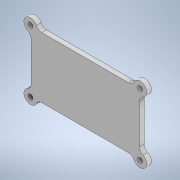
# Autodesk Inventor part: sensor_lid
Saved by Autodesk Inventor 2020 (Build 240168000, 168)
## iProperties
Created: 2020-03-10
Part Number: sensor_lid
Material: Generic
Document SubType Name: Modeling
Designer: Richard
Density: 1 g/cm^3
Appearance: Default
Author: Richard
Autodesk Inventor part; units mm, degrees
ref_plane "YZ Plane" through (0, 0, 0) normal (1, 0, 0) x (0, 1, 0)
sketch "Sketch1" plane through (0, 0, 0) normal (0, 0, 1) x (1, 0, 0)
  line L0 (-172.0273, 68.4234) -> (-119.9573, 68.4234)
  line L1 (-119.9573, 68.4234) -> (-119.9573, 42.0074)
  line L2 (-119.9573, 42.0074) -> (-172.0273, 42.0074)
  line L3 (-172.0273, 42.0074) -> (-172.0273, 68.4234)
  point P0 (0, 0)
  dimension "d0" = 52.07
  dimension "d1" = 26.416
  constraints: 8 end point, 2 parallel, 1 horizontal, 1 perpendicular
  measures "d0" distance of L1.end L2.end
  measures "d1" distance of L0.end L1.end
extrude "Extrusion1" add sketch "Sketch1" along normal blind 2.54
sketch "Sketch2" plane through (0, 0, 2.54) normal (0, 0, 1) x (1, 0, 0)
  line L0 (-119.9573, 68.4234) -> (-172.0273, 68.4234) projected
  line L1 (-119.9573, 68.4234) -> (-172.0273, 68.4234) projected
  line L2 (-172.0273, 68.4234) -> (-172.0273, 42.0074) projected
  line L3 (-172.0273, 42.0074) -> (-119.9573, 42.0074) projected
  line L4 (-119.9573, 42.0074) -> (-119.9573, 68.4234) projected
  line L5 (-116.7823, 38.8324) -> (-175.2023, 38.8324)
  line L6 (-175.2023, 38.8324) -> (-175.2023, 71.5984)
  line L7 (-175.2023, 71.5984) -> (-116.7823, 71.5984)
  line L8 (-116.7823, 71.5984) -> (-116.7823, 38.8324)
  point P0 (0, 0)
  dimension "d18" = 3.175
  dimension "d19" = 3.175
  dimension "d20" = 3.175
  dimension "d21" = 3.175
  dimension "d25" = 32.766
  dimension "d26" = 58.42
  constraints: 8 end point, 2 parallel, 1 horizontal, 1 perpendicular
  measures "d18" distance between parallel lines of L3 L5
  measures "d19" distance between parallel lines of L7 L0
  measures "d20" distance between parallel lines of L4 L8
  measures "d21" distance between parallel lines of L6 L2
  measures "d25" distance between parallel lines of L7 L5
  measures "d26" distance of L5.start L5.end
extrude "Extrusion2" add sketch "Sketch2" along normal blind 2.54 contours L4 L3 L2 L0 | L5 L6 L7 L8
fillet "Fillet1" radius 3.175 4 edges at (-116.7823, 38.8324, 3.81) (-175.2023, 38.8324, 3.81) (-116.7823, 71.5984, 3.81) (-175.2023, 71.5984, 3.81)
sketch "Sketch4" plane through (0, 0, 5.08) normal (0, 0, 1) x (1, 0, 0)
  circle A0 centre (-175.5648, 71.9609) radius 1.3891
  line L0 (-119.9573, 71.5984) -> (-172.0273, 71.5984) projected
  arc A1 (-172.0273, 71.5984) -> (-175.2023, 68.4234) centre (-172.0273, 68.4234) ccw projected
  line L1 (-175.2023, 68.4234) -> (-175.2023, 42.0074) projected
  arc A2 (-172.0273, 71.5984) -> (-175.2023, 68.4234) centre (-175.5648, 71.9609) ccw
  point P0 (0, 0)
  dimension "d12" = 2.7781
  dimension "d23" = 3.556
  constraints: 2 centre point, 2 point on circle, 1 concentric
  measures "d12" diameter of A0
  measures "d23" radius of A2
extrude "Extrusion3" add sketch "Sketch4" against normal up to surface (2.54 mm away)
ref_plane "Work Plane1" through (-145.9923, 42.0074, 2.54) normal (-1, 0, 0) x (0, 0, 1)
ref_plane "Work Plane2" through (-172.0273, 55.2154, 2.54) normal (0, -1, 0) x (1, 0, 0)
mirror "Mirror1" about plane through (-145.9923, 42.0074, 2.54) normal (-1, 0, 0) of "Extrusion3"
mirror "Mirror2" about plane through (-172.0273, 55.2154, 2.54) normal (0, -1, 0) of "Extrusion3", "Mirror1"
fillet "Fillet3" radius 3.175 8 edges at (-175.2023, 42.0074, 3.81) (-175.2023, 68.4234, 3.81) (-119.9573, 38.8324, 3.81) (-172.0273, 71.5984, 3.81) (-119.9573, 71.5984, 3.81) (-116.7823, 68.4234, 3.81) (-116.7823, 42.0074, 3.81) (-172.0273, 38.8324, 3.81)
equation "\"d19\" = d18"
equation "\"d21\" = d20"
body "Solid1"
